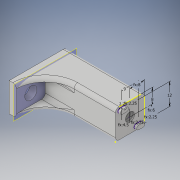
# Autodesk Inventor part: vive_mount
Saved by Autodesk Inventor 2019 (Build 230136000, 136)
## iProperties
Created: 2020-10-08
Part Number: vive_mount
Material: Generic
Document SubType Name: Modeling
Designer: close
Density: 1 g/cm^3
Appearance: Default
Author: close
Autodesk Inventor part; units mm, degrees
ref_plane "YZ Plane" through (0, 0, 0) normal (1, 0, 0) x (0, 1, 0)
ref_plane "XZ Plane" through (0, 0, 0) normal (0, 1, 0) x (-1, 0, 0)
ref_plane "XY Plane" through (0, 0, 0) normal (0, 0, 1) x (1, 0, 0)
sketch "Sketch1" plane through (0, 0, 0) normal (0, 1, 0) x (-1, 0, 0)
  line L0 (43, 16) -> (43, -16)
  line L1 (43, -16) -> (0, -16)
  line L2 (0, -16) -> (0, 0)
  line L3 (0, 0) -> (23, 0)
  line L4 (39, 16) -> (39, 16)
  line L5 (39, 16) -> (43, 16)
  arc A0 (23, 0) -> (39, 16) centre (23, 16) ccw
  dimension "d0" = 16
  dimension "d1" = 32
  dimension "d2" = 4
  dimension "d3" = 16
  dimension "d4" = 43
  constraints: 12 end point, 5 perpendicular, 2 point on circle, 2 tangent, 1 centre point, 1 vertical
  measures "d0" distance between parallel lines of L1 L3
  measures "d1" distance between parallel lines of L1 L5
  measures "d2" distance between parallel lines of L4 L0
  measures "d3" radius of A0
  measures "d4" distance between parallel lines of L2 L0
extrude "Extrusion1" add sketch "Sketch1" along normal blind 16
fillet "Fillet1" radius 2 6 edges at (-34.3137, 16, 4.6863) (-11.5, 16, 0) (-21.5, 16, -16) (-21.5, 0, -16) (-34.3137, 0, 4.6863) (-11.5, 0, 0)
ref_plane "Work Plane1" through (-39, 0, 16) normal (-1, 0, 0) x (0, 0, 1)
sketch "Sketch2" plane through (-39, 0, 16) normal (-1, 0, 0) x (0, 0, 1)
  line L0 (-16, 14) -> (0, 14) projected
  line L1 (0, 2) -> (-16, 2) projected
  line L2 (-14, 14) -> (0, 14)
  line L3 (0, 14) -> (0, 2)
  line L4 (0, 2) -> (-14, 2)
  line L5 (-16, 4) -> (-16, 12)
  arc A0 (-14, 14) -> (-16, 12) centre (-14, 12) ccw
  arc A1 (-16, 4) -> (-14, 2) centre (-14, 4) ccw
  point P0 (-16, 0)
  dimension "d9" = 2
  dimension "d10" = 16
  constraints: 8 end point, 4 point on circle, 4 tangent, 3 point on line, 2 centre point, 2 parallel, 1 equal radius, 1 horizontal, 1 perpendicular
  measures "d9" radius of A0
  measures "d10" distance between parallel lines of L3 L5
extrude "Extrusion2" cut sketch "Sketch2" against normal blind 16
sketch "Sketch3" plane through (-39, 0, 16) normal (1, 0, 0) x (0, 0, -1)
  line L0 (0, 0) -> (18, 0) projected
  line L1 (18, 16) -> (0, 16) projected
  line L2 (0, 2) -> (0, 14) projected
  point P0 (16, 0)
  point P1 (8, 8)
  dimension "d13" = 16
  dimension "d14" = 8
  dimension "d15" = 8
  measures "d13" distance between parallel lines of L0 L1
  measures "d14" distance from line of L1 point (8, 8)
  measures "d15" distance from line of L2 point (8, 8)
hole "Hole1" at (-39, 8, 8) direction (-1, 0, 0) diameter 6.756 depth 8.8 clearance for "Flat Head Machine Screw (82)" size "1/4" standard "Ansi Unified Screw Threads"
sketch "Sketch4" plane through (0, 0, -2) normal (1, 0, 0) x (0, 0, -1)
  line L0 (0, 16) -> (12, 16) projected
  line L1 (14, 2) -> (14, 14) projected
  line L2 (0.375, 14) -> (2.625, 14) construction
  line L3 (0.375, 12.875) -> (2.625, 12.875)
  line L4 (2.625, 15.125) -> (0.375, 15.125)
  arc A0 (0.375, 15.125) -> (0.375, 12.875) centre (0.375, 14) ccw
  arc A1 (2.625, 12.875) -> (2.625, 15.125) centre (2.625, 14) ccw
  line L5 (9.375, 2) -> (11.625, 2) construction
  line L6 (9.375, 0.875) -> (11.625, 0.875)
  line L7 (11.625, 3.125) -> (9.375, 3.125)
  arc A2 (9.375, 3.125) -> (9.375, 0.875) centre (9.375, 2) ccw
  arc A3 (11.625, 0.875) -> (11.625, 3.125) centre (11.625, 2) ccw
  point P0 (-2, 0)
  point P1 (6, 8)
  point P2 (1.5, 14)
  point P3 (10.5, 2)
  dimension "d23" = 8
  dimension "d24" = 8
  dimension "d25" = 9
  dimension "d26" = 4.5
  dimension "d27" = 2.25
  dimension "d28" = 2.25
  dimension "d29" = 2.25
  dimension "d30" = 2.25
  dimension "d31" = 12
  dimension "d32" = 6
  constraints: 16 end point, 8 point on circle, 8 tangent, 4 centre point, 3 parallel, 2 midpoint, 1 horizontal
  measures "d23" distance from line of L0 point (6, 8)
  measures "d24" distance from line of L1 point (6, 8)
  measures "d25" horizontal distance of point (10.5, 2) point (1.5, 14)
  measures "d26" horizontal distance of point (6, 8) point (1.5, 14)
  measures "d27" distance of L2.start L2.end
  measures "d28" distance between parallel lines of L3 L4
  measures "d29" distance between parallel lines of L6 L7
  measures "d30" distance of L7.start L7.end
  measures "d31" vertical distance of point (1.5, 14) point (10.5, 2)
  measures "d32" vertical distance of point (6, 8) point (10.5, 2)
extrude "Extrusion3" add sketch "Sketch4" along normal blind 1.5
hole "Hole2" at (0, 8, -8) direction (-1, 0, 0) diameter 4.978 depth 19.05 thread size "1/4-20 UNC" class "2B" standard "ANSI Unified Screw Threads"
equation "\"d1\" = 2 * d0"
equation "\"d14\" = 0.5 * d13"
equation "\"d15\" = 0.5 * d13"
equation "\"d24\" = d23"
equation "\"d26\" = 0.5 * d25"
equation "\"d28\" = d27"
equation "\"d29\" = d28"
equation "\"d30\" = d29"
equation "\"d32\" = 0.5 * d31"
body "Solid1"
